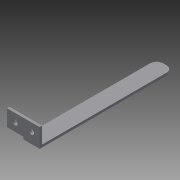
# Autodesk Inventor part: Fork 1 right ver2
Saved by Autodesk Inventor 2015 (Build 190159000, 159)
## iProperties
Created: 2015-06-20
Part Number: Fork 1 right ver2
Material: アルミニウム 5052 H32
Document SubType Name: Modeling
Designer: kenta
Density: 2.68 g/cm^3
Appearance: サテン
Mass: 3.99201 g
Surface Area: 23.4464 cm^2
Volume: 1.48956 cm^3
Author: kenta
Autodesk Inventor part; units mm, degrees
ref_plane "YZ Plane" through (0, 0, 0) normal (1, 0, 0) x (0, 1, 0)
ref_plane "XZ Plane" through (0, 0, 0) normal (0, 1, 0) x (-1, 0, 0)
ref_plane "XY Plane" through (0, 0, 0) normal (0, 0, 1) x (1, 0, 0)
sketch "スケッチ1" plane through (0, 0, 0) normal (0, 0, 1) x (1, 0, 0)
  line L0 (0, 0) -> (10, 0)
  line L1 (10, 0) -> (10, -80)
  line L2 (10, -80) -> (0, -80)
  line L3 (0, -80) -> (0, 0)
  dimension "d0" = 10
  dimension "d1" = 80
  constraints: 8 end point, 2 parallel, 1 horizontal, 1 perpendicular
  measures "d0" distance of L1.end L2.end
  measures "d1" distance of L0.end L1.end
extrude "押し出し1" add sketch "スケッチ1" along normal blind 1.5
fillet "フィレット1" radius 4 2 edges at (10, 0, 0.75) (0, 0, 0.75)
sketch "スケッチ2" plane through (0, -80, 0) normal (0, -1, 0) x (1, 0, 0)
  line L0 (0, 1.5) -> (10, 1.5)
  line L1 (10, 1.5) -> (10, 0)
  line L2 (10, 0) -> (0, 0)
  line L3 (0, 0) -> (0, 1.5)
  constraints: 8 end point, 2 parallel, 1 horizontal, 1 perpendicular
extrude "押し出し2" add sketch "スケッチ2" along normal blind 1.5
sketch "スケッチ4" plane through (0, 0, 1.5) normal (0, 0, 1) x (1, 0, 0)
  line L0 (20, -81.5) -> (-10, -81.5)
  line L1 (-10, -81.5) -> (-10, -80)
  line L2 (-10, -80) -> (20, -80)
  line L3 (20, -80) -> (20, -81.5)
  point P0 (0, 0)
  dimension "d10" = 30
  dimension "d11" = 1.5
  constraints: 8 end point, 2 parallel, 1 horizontal, 1 perpendicular
  measures "d10" distance of L1.end L2.end
  measures "d11" distance of L0.end L1.end
extrude "押し出し4" add sketch "スケッチ4" along normal blind 10
sketch "スケッチ5" plane through (-10, -80, 1.5) normal (0, 1, 0) x (1, 0, 0)
  line L0 (30, -10) -> (20, -10)
  line L1 (20, -10) -> (20, 0)
  line L2 (20, 0) -> (30, 0)
  line L3 (30, 0) -> (30, -10)
  point P0 (10, 1.5)
  dimension "d14" = 10
  dimension "d15" = 10
  constraints: 8 end point, 2 parallel, 1 horizontal, 1 perpendicular
  measures "d14" distance of L1.end L2.end
  measures "d15" distance of L0.end L1.end
extrude "押し出し5" cut sketch "スケッチ5" against normal blind 10
sketch "スケッチ7" plane through (-10, -80, 1.5) normal (0, 1, 0) x (1, 0, 0)
  line L0 (20, -10) -> (0, -10) projected
  line L1 (20, -10) -> (20, 0) projected
  point P0 (10, 1.5)
  point P1 (15, -5)
  point P2 (5, -5)
  dimension "d23" = 10
  dimension "d24" = 5
  dimension "d25" = 5
  constraints: 1 horizontal alignment
  measures "d23" distance of point (5, -5) point (15, -5)
  measures "d24" distance from line of point (15, -5) L0
  measures "d25" distance from line of point (15, -5) L1
hole "穴1" at (5, -80, 6.5) at (-5, -80, 6.5) direction (0, -1, 0) diameter 3.1 depth 8 tip angle 118
